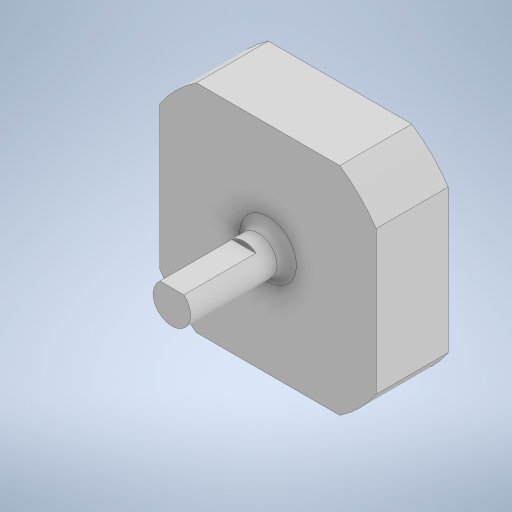
# Autodesk Inventor part: 손잡이 축
Saved by Autodesk Inventor 2023 (Build 270158000, 158)
## iProperties
Created: 2022-06-24
Part Number: 손잡이 축
Material: 일반
Document SubType Name: Modeling
Designer: user
Density: 1 g/cm^3
Appearance: 기본값
Author: user
Autodesk Inventor part; units mm, degrees
ref_plane "YZ Plane" through (0, 0, 0) normal (1, 0, 0) x (0, 1, 0)
ref_plane "XZ Plane" through (0, 0, 0) normal (0, 1, 0) x (-1, 0, 0)
ref_plane "XY Plane" through (0, 0, 0) normal (0, 0, 1) x (1, 0, 0)
sketch "스케치1" plane through (0, 0, 0) normal (0, 0, 1) x (1, 0, 0)
  circle A0 centre (0, 0) radius 27
  line L0 (-22.5, -22.5) -> (22.5, -22.5)
  line L1 (22.5, -22.5) -> (22.5, 22.5)
  line L2 (22.5, 22.5) -> (-22.5, 22.5)
  line L3 (-22.5, 22.5) -> (-22.5, -22.5)
  line L4 (-22.5, -22.5) -> (22.5, 22.5) construction
  line L5 (22.5, -22.5) -> (-22.5, 22.5) construction
  point P0 (-22.5, 14.9248)
  point P1 (-22.5, -14.9248)
  point P2 (-14.9248, -22.5)
  point P3 (14.9248, -22.5)
  point P4 (22.5, -14.9248)
  point P5 (22.5, 14.9248)
  point P6 (14.9248, 22.5)
  point P7 (-14.9248, 22.5)
  dimension "d0" = 54
  dimension "d5" = 45
  dimension "d6" = 45
  constraints: 12 end point, 2 midpoint, 2 parallel, 1 centre point, 1 coincident, 1 horizontal, 1 perpendicular
  measures "d0" diameter of A0
  measures "d5" distance of L2.end L1.end
  measures "d6" distance of L1.end L0.end
extrude "돌출1" add sketch "스케치1" along normal blind 15 contours L1 A0 L0 L3 L2
sketch "스케치2" plane through (0, 0, 15) normal (0, 0, 1) x (1, 0, 0)
  point P0 (0, 0)
sketch "스케치3" plane through (0, 0, 15) normal (0, 0, 1) x (1, 0, 0)
  circle A0 centre (0, 0) radius 3.9
  line L0 (-2.492, 3) -> (2.492, 3)
  dimension "d7" = 7.8
  dimension "d8" = 3
  constraints: 2 end point, 2 point on circle, 1 centre point, 1 coincident, 1 horizontal
  measures "d7" diameter of A0
  measures "d8" distance from line of point (0, 0) L0
extrude "돌출2" add sketch "스케치3" along normal blind 20 contours A0 L0 picked at (1.186, -0.6989)
extrude "돌출3" add sketch "스케치3" along normal blind 5 contours L0 A0 picked at (-0.5796, 3.1636)
fillet "모깎기1" radius 2 1 edges at (-2.492, -3, 15)
